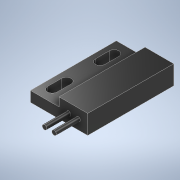
# Autodesk Inventor part: 59145_Sensor
Saved by Autodesk Inventor 2021 (Build 250183000, 183)
## iProperties
Created: 2021-10-07
Part Number: 59145_Sensor
Material: Generic
Document SubType Name: Modeling
Designer: Jorian Brusind
Density: 1 g/cm^3
Appearance: Glossy - Black
Author: Jorian Brusind
Autodesk Inventor part; units mm, degrees
ref_plane "YZ Plane" through (0, 0, 0) normal (1, 0, 0) x (0, 1, 0)
ref_plane "XZ Plane" through (0, 0, 0) normal (0, 1, 0) x (-1, 0, 0)
ref_plane "XY Plane" through (0, 0, 0) normal (0, 0, 1) x (1, 0, 0)
sketch "Sketch1" plane through (0, 0, 0) normal (0, 1, 0) x (-1, 0, 0)
  line L0 (0, 0) -> (19.05, 0)
  line L1 (19.05, 0) -> (19.05, -28.57)
  line L2 (19.05, -28.57) -> (0, -28.57)
  line L3 (0, -28.57) -> (0, 0)
  dimension "d0" = 19.05
  dimension "d1" = 28.57
  constraints: 8 end point, 2 parallel, 1 horizontal, 1 perpendicular
  measures "d0" distance of L1.end L2.end
  measures "d1" distance of L0.end L1.end
extrude "Extrusion1" add sketch "Sketch1" along normal blind 3.43
sketch "Sketch2" plane through (0, 3.43, 0) normal (0, 1, 0) x (1, 0, 0)
  line L0 (0, 28.57) -> (-19.05, 28.57) projected
  line L1 (0, 0) -> (-9.53, 0)
  line L2 (-9.53, 0) -> (-9.53, 28.57)
  line L3 (-9.53, 28.57) -> (0, 28.57)
  line L4 (0, 28.57) -> (0, 0)
  dimension "d4" = 9.53
  constraints: 8 end point, 2 parallel, 1 horizontal, 1 perpendicular, 1 point on line
  measures "d4" distance of L2.end L3.end
extrude "Extrusion2" add sketch "Sketch2" along normal blind 2.92
sketch "Sketch3" plane through (0, 6.35, 0) normal (0, 1, 0) x (1, 0, 0)
  line L0 (-15.75, 4.02) -> (-15.75, 8.66) construction
  line L1 (-14.16, 4.02) -> (-14.16, 8.66)
  line L2 (-17.34, 8.66) -> (-17.34, 4.02)
  arc A0 (-17.34, 4.02) -> (-14.16, 4.02) centre (-15.75, 4.02) ccw
  arc A1 (-14.16, 8.66) -> (-17.34, 8.66) centre (-15.75, 8.66) ccw
  line L3 (-19.05, 28.57) -> (-19.05, 0) projected
  line L4 (-15.75, 19.9) -> (-15.75, 24.54) construction
  line L5 (-14.16, 19.9) -> (-14.16, 24.54)
  line L6 (-17.34, 24.54) -> (-17.34, 19.9)
  arc A2 (-17.34, 19.9) -> (-14.16, 19.9) centre (-15.75, 19.9) ccw
  arc A3 (-14.16, 24.54) -> (-17.34, 24.54) centre (-15.75, 24.54) ccw
  line L7 (0, 28.57) -> (-9.53, 28.57) projected
  point P0 (0, 0)
  point P1 (-15.75, 6.34)
  point P2 (-15.75, 22.22)
  dimension "d7" = 4.64
  dimension "d8" = 3.18
  dimension "d9" = 3.3
  dimension "d10" = 4.64
  dimension "d11" = 3.18
  dimension "d12" = 15.88
  dimension "d13" = 6.35
  constraints: 16 end point, 8 point on circle, 8 tangent, 4 centre point, 2 midpoint, 2 parallel, 2 vertical
  measures "d7" distance of L0.start L0.end
  measures "d8" diameter of A1
  measures "d9" distance from line of L3 point (-15.75, 6.34)
  measures "d10" distance of L4.start L4.end
  measures "d11" diameter of A3
  measures "d12" distance of point (-15.75, 22.22) point (-15.75, 6.34)
  measures "d13" distance from line of L7 point (-15.75, 22.22)
extrude "Extrusion3" cut sketch "Sketch3" against normal through all
sketch "Sketch4" plane through (-19.05, 0, 0) normal (0, 0, 1) x (1, 0, 0)
  line L0 (9.52, 6.35) -> (19.05, 6.35) projected
  line L1 (9.52, 6.35) -> (12.69, 6.35)
  line L2 (12.69, 6.35) -> (12.69, 0)
  line L3 (0, 0) -> (19.05, 0) projected
  line L4 (19.05, 0) -> (19.05, 6.35) projected
  line L5 (19.05, 6.35) -> (15.87, 6.35)
  line L6 (15.87, 6.35) -> (15.87, 0)
  circle A0 centre (12.69, 3.175) radius 0.75
  circle A1 centre (15.87, 3.175) radius 0.75
  dimension "d20" = 3.17
  dimension "d21" = 3.18
  dimension "d24" = 1.5
  dimension "d25" = 1.5
  constraints: 8 end point, 2 centre point, 2 midpoint, 2 perpendicular, 2 point on line, 1 collinear, 1 horizontal
  measures "d20" distance of L0.start L1.end
  measures "d21" distance of L0.end L5.end
  measures "d24" diameter of A0
  measures "d25" diameter of A1
extrude "Extrusion4" add sketch "Sketch4" along normal blind 8 contours A0 L2 | L2 A0 | A1 L6 | L6 A1
body "Solid1"
